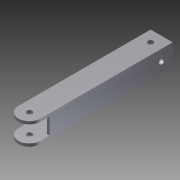
# Autodesk Inventor part: pnumatic arm lever
Saved by Autodesk Inventor 2012 (Build 160160000, 160)
## iProperties
Created: 2013-09-06
Part Number: pnumatic arm lever
Material: Default
Document SubType Name: Modeling
Designer: Bryce
Density: 1 g/cm^3
Author: Bryce
Autodesk Inventor part; units mm, degrees
ref_plane "YZ Plane" through (0, 0, 0) normal (1, 0, 0) x (0, 1, 0)
ref_plane "XZ Plane" through (0, 0, 0) normal (0, 1, 0) x (-1, 0, 0)
ref_plane "XY Plane" through (0, 0, 0) normal (0, 0, 1) x (1, 0, 0)
sketch "Sketch1" plane through (0, 0, 0) normal (0, 0, 1) x (1, 0, 0)
  line L0 (0, 0) -> (25.4, 0)
  line L1 (25.4, 0) -> (25.4, 25.4)
  line L2 (25.4, 25.4) -> (0, 25.4)
  line L3 (0, 25.4) -> (0, 0)
  line L4 (3.175, 3.175) -> (22.225, 3.175)
  line L5 (22.225, 3.175) -> (22.225, 22.225)
  line L6 (22.225, 22.225) -> (3.175, 22.225)
  line L7 (3.175, 22.225) -> (3.175, 3.175)
  dimension "d0" = 3.175
  dimension "d1" = 3.175
  dimension "d2" = 3.175
  dimension "d3" = 3.175
  dimension "d4" = 25.4
  dimension "d5" = 25.4
  constraints: 16 end point, 4 parallel, 2 horizontal, 2 perpendicular
  measures "d0" distance between parallel lines of L2 L6
  measures "d1" distance between parallel lines of L1 L5
  measures "d2" distance between parallel lines of L0 L4
  measures "d3" distance between parallel lines of L3 L7
  measures "d4" distance of L2.end L0.start
  measures "d5" distance of L0.start L0.end
extrude "Extrusion1" add sketch "Sketch1" along normal blind 165.1
sketch "Sketch2" plane through (0, 25.4, 0) normal (0, 1, 0) x (1, 0, 0)
  line L0 (0, -165.1) -> (25.4, -165.1) projected
  line L1 (25.4, 0) -> (25.4, -165.1) projected
  line L2 (25.4, 0) -> (0, 0) projected
  line L3 (0, 0) -> (0, -165.1) projected
  circle A0 centre (12.7, -152.4) radius 3.175
  arc A1 (0, -152.4) -> (25.4, -152.4) centre (12.7, -152.4) ccw
  circle A2 centre (12.7, -12.7) radius 3.175
  point P0 (12.7, 0)
  dimension "d8" = 6.35
  dimension "d17" = 12.7
  dimension "d18" = 6.35
  constraints: 3 centre point, 3 tangent, 2 point on circle, 2 point on line, 1 coincident, 1 midpoint, 1 vertical alignment
  measures "d8" diameter of A0
  measures "d17" distance from line of L2 A2.centre
  measures "d18" diameter of A2
extrude "Extrusion2" cut sketch "Sketch2" against normal through all contours L3 A1 L0 | A1 L1 L0 | A0 | A2
sketch "Sketch3" plane through (25.4, 0, 0) normal (1, 0, 0) x (0, 0, -1)
  line L0 (0, 0) -> (0, 25.4) projected
  line L1 (0, 25.4) -> (-152.4, 25.4) projected
  line L2 (-160.8003, 3.175) -> (-160.8003, 22.225) projected
  line L3 (-160.8003, 22.225) -> (-141.7503, 22.225)
  line L4 (-141.7503, 22.225) -> (-141.7503, 3.175)
  line L5 (-141.7503, 3.175) -> (-160.8003, 3.175)
  line L6 (-160.8003, 3.175) -> (-160.8003, 22.225)
  circle A0 centre (-12.7, 12.7) radius 3.175
  dimension "d11" = 19.05
  dimension "d12" = 6.35
  dimension "d13" = 12.7
  dimension "d14" = 12.7
  constraints: 8 end point, 2 parallel, 1 centre point, 1 horizontal, 1 perpendicular
  measures "d11" distance of L2.end L3.end
  measures "d12" diameter of A0
  measures "d13" distance from line of L0 A0.centre
  measures "d14" distance from line of L1 A0.centre
extrude "Extrusion3" cut sketch "Sketch3" against normal through all
equation "\"d0\" = d3"
equation "\"d1\" = d3"
equation "\"d2\" = d1"
equation "\"d18\" = d8"
body "Solid1"
